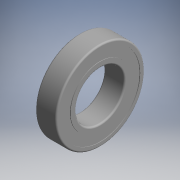
# Autodesk Inventor part: bearing_6006
Saved by Autodesk Inventor 2017.3 (Build 213256000, 256)
## iProperties
Part Number: bearing_6006
Material: Generic
Catalog Web Link: www.cadenas.de
Description: 6000_bearing-Deep Groove Ball Bearings
Vendor: MISUMI
Document SubType Name: Modeling
Designer: partserver
Manufacturer: MISUMI
Mass: 21.0144 g
Surface Area: 67.6627 cm^2
Volume: 21.0144 cm^3
Density: 1 g/cm^3
Appearance: PSOLRGB-192-192-192
Category: PARTsolutions
Company: MISUMI
Title: bearing_6006
Author: Cadenas PARTsolutions
Comments: Deep Groove Ball Bearings
PSOL_IDENT_0: {$CADENAS_DATA\23d-libs\misumi\metric\accessories\bearing_6000.prj},171 {VTYP=3D},{NB=bearing_6006},
PSOL_IDENT_1: {LINA=bearing_6006},{NN=6000_bearing},{DATE=30.10.2020 15:47:11},{GEOMDATE=24.10.2013 00:00:00},{VER
PSOL_IDENT_2: SION=},{LINEID=310},{WBVAR=},{WBNUMERIC=}  {NB=bearing_6006},{LINA=bearing_6006},{KT=DUMMY},{PN=bear
PSOL_IDENT_3: ing_6006},{BN=6006},{DD=30},{D=55},{B=13},{RR=1.0},{DSMIN=35.0},{DS1=37.00},{DSMAX=37.00},{DDHH=50.0
PSOL_IDENT_4: },{R=1.0},{R1=0.400},{R2=1.000},{MASS=116},{MASS11=116},{AA=12.3160},{BB=2.8000},{CC=3.6000},{DD1=52
PSOL_IDENT_5: .600}
NB: bearing_6006
NN: 6000_bearing
NT: Deep Groove Ball Bearings
NBSYN: $PN.
LINA: bearing_6006
CATALOG: Misumi
PN: bearing_6006
BN: 6006
DD: 30
D: 55
B: 13
RR: 1
DSMIN: 35
DDHH: 50
R: 1
MASS11: 116
SUPPLIER: MISUMI
ARTICLENO: bearing_6006
BOMINFO: bearing_6006
CREATOR: CADENAS GmbH
Autodesk Inventor part; units mm, degrees
sketch "Sketch_1" plane through (0, 0, 0) normal (0, 0, 1) x (1, 0, 0)
  line L0 (13, 0) -> (0, 0)
  arc A0 (0, 16) -> (1, 15) centre (1, 16) ccw
  line L1 (1, 15) -> (12, 15)
  arc A1 (12, 15) -> (13, 16) centre (12, 16) ccw
  line L2 (13, 16) -> (13, 18.6)
  line L3 (13, 18.6) -> (12.658, 18.6)
  line L4 (12.658, 18.6) -> (12.658, 24.7)
  line L5 (12.658, 24.7) -> (13, 24.7)
  line L6 (13, 24.7) -> (13, 26.5)
  arc A2 (13, 26.5) -> (12, 27.5) centre (12, 26.5) ccw
  line L7 (12, 27.5) -> (1, 27.5)
  arc A3 (1, 27.5) -> (0, 26.5) centre (1, 26.5) ccw
  line L8 (0, 26.5) -> (0, 24.7)
  line L9 (0, 24.7) -> (0.342, 24.7)
  line L10 (0.342, 24.7) -> (0.342, 18.6)
  line L11 (0.342, 18.6) -> (0, 18.6)
  line L12 (0, 18.6) -> (0, 16)
  constraints: 26 end point, 8 point on circle, 4 centre point
revolve "Revolution1" add sketch "Sketch_1" angle 360 about axis through (13, 0, 0) along (1, 0, 0)
ref_plane "center_point_XY" through (6.5, 0, 0) normal (1, 0, 0) x (0, 0, -1)
ref_plane "center_point_YZ" through (6.5, 0, 0) normal (0, 0, -1) x (0, 1, 0)
ref_plane "center_point_ZX" through (6.5, 0, 0) normal (0, 1, 0) x (1, 0, 0)
ref_plane "to_housing_XY" through (0, 0, 0) normal (1, 0, 0) x (0, 0, -1)
ref_plane "to_housing_YZ" through (0, 0, 0) normal (0, 0, -1) x (0, 1, 0)
ref_plane "to_housing_ZX" through (0, 0, 0) normal (0, 1, 0) x (1, 0, 0)
ref_plane "to_ring_XY" through (12.316, 0, 0) normal (1, 0, 0) x (0, 0, -1)
ref_plane "to_ring_YZ" through (12.316, 0, 0) normal (0, 0, -1) x (0, 1, 0)
ref_plane "to_ring_ZX" through (12.316, 0, 0) normal (0, 1, 0) x (1, 0, 0)
body "Solid1"
